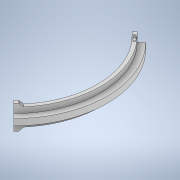
# Autodesk Inventor part: BinnenringMiddenStuk
Saved by Autodesk Inventor 2022 (Build 260153000, 153)
## iProperties
Created: 2022-04-04
Part Number: BinnenringMiddenStuk
Material: Generic
Document SubType Name: Modeling
Designer: Seppe
Density: 1 g/cm^3
Appearance: Default
Author: Seppe
Autodesk Inventor part; units mm, degrees
ref_plane "YZ Plane" through (0, 0, 0) normal (1, 0, 0) x (0, 1, 0)
sketch "Sketch1" plane through (0, 0, 0) normal (0, 1, 0) x (-1, 0, 0)
  circle A0 centre (0, 0) radius 124.6
  circle A1 centre (0, 0) radius 114.6
  line L0 (0, -124.6) -> (0, 124.6)
  point P0 (0, 114.6)
  point P1 (0, -114.6)
  dimension "d88" = 249.2
  dimension "d89" = 229.2
  constraints: 2 centre point, 2 end point, 2 point on circle, 1 coincident, 1 vertical
  measures "d88" diameter of A0
  measures "d89" diameter of A1
extrude "Extrusion18" add sketch "Sketch1" along normal mid plane 25 contours L0 A1 A0 picked at (-5.2055, 120.9392)
sketch "Sketch21" plane through (0, 0, 0) normal (0, 1, 0) x (-1, 0, 0)
  circle A0 centre (0, 0) radius 124.6
  circle A1 centre (0, 0) radius 133.25
  line L0 (0, -133.25) -> (0, 133.25)
  point P0 (0, -124.6)
  point P1 (0, 124.6)
  dimension "d92" = 266.5
  constraints: 2 centre point, 2 coincident, 2 end point, 2 point on circle, 1 vertical
  measures "d92" diameter of A1
extrude "Extrusion19" add sketch "Sketch21" along normal mid plane 9 contours A0 L0 A1 picked at (-127.3194, 0)
ref_plane "Work Plane2" through (0, 0, -114.6) normal (0, 0, 1) x (1, 0, 0)
sketch "Sketch23" plane through (0, 0, -114.6) normal (0, 0, 1) x (1, 0, 0)
  line L0 (0, 17.5) -> (6.5, 17.5)
  line L1 (6.5, 17.5) -> (6.5, -17.5)
  line L2 (6.5, -17.5) -> (0, -17.5)
  line L3 (0, -17.5) -> (0, 17.5)
  line L4 (0, -12.5) -> (0, 12.5) projected
  point P0 (0, 0)
  point P1 (0, 8)
  dimension "d98" = 6.5
  dimension "d99" = 35
  dimension "d100" = 0
  dimension "d101" = 17.5
  constraints: 8 end point, 2 parallel, 1 horizontal, 1 perpendicular
  measures "d98" distance of L1.end L2.end
  measures "d99" distance of L0.end L1.end
  measures "d100" distance between parallel lines of L4 L3
  measures "d101" distance from line of point (0, 0) L0
extrude "Extrusion21" add sketch "Sketch23" against normal blind 10
sketch "Sketch25" plane through (0, 0, 0) normal (0, 1, 0) x (-1, 0, 0)
  line L0 (0, -114.6) -> (-11.5, -114.6)
  line L1 (-11.5, -114.6) -> (-11.5, -104.6)
  line L2 (-11.5, -104.6) -> (0, -104.6)
  line L3 (0, -104.6) -> (0, -114.6)
  point P0 (0, 0)
  dimension "d104" = 11.5
  dimension "d105" = 10
  constraints: 8 end point, 2 parallel, 1 horizontal, 1 perpendicular
  measures "d104" distance of L1.end L2.end
  measures "d105" distance of L0.end L1.end
extrude "Extrusion22" cut sketch "Sketch25" along normal through all both and the other way through all
ref_plane "Work Plane3" through (0, 17.5, -119.6) normal (0, 0, -1) x (1, 0, 0)
sketch "Sketch26" plane through (0, 17.5, -119.6) normal (0, 0, -1) x (1, 0, 0)
  circle A0 centre (0, 17.5) radius 13
  dimension "d108" = 26
  constraints: 1 centre point, 1 coincident
  measures "d108" diameter of A0
extrude "Extrusion23" cut sketch "Sketch26" along normal mid plane 6
sketch "Sketch27" plane through (0, 17.5, -119.6) normal (0, 0, -1) x (1, 0, 0)
  circle A0 centre (0, 17.5) radius 8
  dimension "d111" = 16
  constraints: 1 centre point, 1 coincident
  measures "d111" diameter of A0
extrude "Extrusion24" cut sketch "Sketch27" along normal through all both and the other way through all
sketch "Sketch28" plane through (0, 4.5, 0) normal (0, 1, 0) x (1, 0, 0)
  line L0 (6.6144, 133.0857) -> (6.6144, 124.4243) projected
  circle A0 centre (33.7757, 0) radius 127.3544
  circle A1 centre (0, 0) radius 168.1211
  line L1 (-168.1211, 0) -> (168.1211, 0)
  line L2 (6.6144, 124.4243) -> (6.6144, 167.991)
  point P0 (161.1301, 0)
  constraints: 4 end point, 3 point on circle, 1 centre point, 1 coincident, 1 horizontal, 1 point on line, 3 other
extrude "Extrusion25" cut sketch "Sketch28" along normal through all both and the other way through all contours L2 A1 L1 A0 L0 picked at (33.6565, 152.3073)
sketch "Sketch29" plane through (0, 17.5, -124.6) normal (-1, 0, 0) x (0, 0, 1)
  circle A0 centre (2.5, -2.5) radius 1
  circle A1 centre (7.5, -2.5) radius 1
  circle A2 centre (2.5, -32.5) radius 1
  circle A3 centre (7.5, -32.5) radius 1
  line L0 (0, -9.5) -> (0, 0) projected
  line L1 (10, 0) -> (0, 0) projected
  line L2 (10, -9.5) -> (10, 0) projected
  line L3 (10, -35) -> (0, -35) projected
  line L4 (0, -35) -> (0, -25.5) projected
  line L5 (10, -35) -> (10, -25.5) projected
  point P0 (124.6, -17.5)
  dimension "d119" = 2
  dimension "d120" = 2
  dimension "d121" = 2
  dimension "d122" = 2
  dimension "d123" = 2.5
  dimension "d124" = 2.5
  dimension "d125" = 2.5
  dimension "d126" = 2.5
  dimension "d127" = 2.5
  dimension "d128" = 2.5
  dimension "d129" = 2.5
  dimension "d130" = 2.5
  constraints: 4 centre point
  measures "d119" diameter of A0
  measures "d120" diameter of A1
  measures "d121" diameter of A2
  measures "d122" diameter of A3
  measures "d123" distance from line of L0 A0.centre
  measures "d124" distance from line of L1 A0.centre
  measures "d125" distance from line of L1 A1.centre
  measures "d126" distance from line of L2 A1.centre
  measures "d127" distance from line of L3 A2.centre
  measures "d128" distance from line of L4 A2.centre
  measures "d129" distance from line of L3 A3.centre
  measures "d130" distance from line of L5 A3.centre
extrude "Extrusion26" cut sketch "Sketch29" against normal blind 6.5
sketch "Sketch31" plane through (0, 0, -124.6) normal (0, 0, -1) x (-1, 0, 0)
  line L0 (-6.5, 17.5) -> (-6.5, 4.6637) projected
  line L1 (-6.5, 12.5) -> (-11.5, 12.5) projected
  line L2 (-6.5, 17.5) -> (-11.5, 17.5)
  line L3 (-11.5, 17.5) -> (-11.5, 12.5)
  line L4 (-11.5, 12.5) -> (-6.5, 12.5)
  line L5 (-6.5, 12.5) -> (-6.5, 17.5)
  line L6 (-11.5, 12.5) -> (-6.5, 17.5)
  point P0 (0, 0)
  constraints: 10 end point, 2 parallel, 1 horizontal, 1 perpendicular
extrude "Extrusion28" add sketch "Sketch31" against normal blind 10 contours L0 L1 L6
sketch "Sketch33" plane through (6.5, 15, -122.1) normal (-1, 0, 0) x (0, 0, 1)
  circle A0 centre (0, 0) radius 2
  circle A1 centre (5, 0) radius 1 projected
  circle A2 centre (5, 0) radius 2
  circle A3 centre (0, -30) radius 1 projected
  circle A4 centre (0, -30) radius 2
  circle A5 centre (5, -30) radius 1 projected
  circle A6 centre (5, -30) radius 2
  point P0 (122.1, -15)
  dimension "d137" = 4
  dimension "d138" = 4
  dimension "d139" = 4
  dimension "d140" = 4
  constraints: 4 centre point, 3 coincident
  measures "d137" diameter of A0
  measures "d138" diameter of A2
  measures "d139" diameter of A4
  measures "d140" diameter of A6
extrude "Extrusion29" cut sketch "Sketch33" against normal blind 10 contours A0 | A1 | A2 | A3 | A4 | A5 | A6
sketch "Sketch34" plane through (0, 12.5, 0) normal (0, 1, 0) x (1, 0, 0)
  circle A0 centre (0, 0) radius 124.6
  circle A1 centre (0, 0) radius 133.25
  constraints: 2 centre point, 2 coincident
extrude "Extrusion30" cut sketch "Sketch34" along normal blind 5 and the other way blind 8
mirror "Mirror1" about plane through (0, 0, 0) normal (0, 1, 0) of "Extrusion29", "Extrusion26", "Extrusion28"
sketch "Sketch35" plane through (0, -12.5, 0) normal (0, -1, 0) x (1, 0, 0)
  circle A0 centre (0, 0) radius 124.6
  arc A1 (11.5, -124.0682) -> (0, 124.6) centre (0, 0) ccw projected
  circle A2 centre (0, 0) radius 127.0013
  constraints: 2 centre point, 2 coincident
extrude "Extrusion31" cut sketch "Sketch35" along normal blind 5 and the other way blind 8
mirror "Mirror2" about plane through (0, 0, 0) normal (0, 0, 1) of "Extrusion29", "Extrusion28", "Extrusion21", "Extrusion24", "Extrusion23", "Extrusion26"
mirror "Mirror3" about plane through (0, 0, 0) normal (0, 0, 1) of "Extrusion25"
mirror "Mirror4" about plane through (0, 0, 0) normal (0, 0, 1) of "Extrusion30"
sketch "Sketch37" plane through (0, 12.5, 0) normal (0, 1, 0) x (1, 0, 0)
  line L0 (6.5, -114.6) -> (0, -114.6) projected
  line L1 (0, -114.6) -> (11.5, -114.6)
  line L2 (11.5, -114.6) -> (11.5, -107.0167)
  line L3 (11.5, -107.0167) -> (0, -107.0167)
  line L4 (0, -107.0167) -> (0, -114.6)
  point P0 (0, 0)
  constraints: 8 end point, 2 parallel, 1 horizontal, 1 perpendicular
extrude "Extrusion32" cut sketch "Sketch37" against normal through all
sketch "Sketch42" plane through (0, 12.5, 0) normal (0, 1, 0) x (1, 0, 0)
  line L0 (0, 0) -> (94.222, -94.222)
  arc A0 (39.6322, -127.2197) -> (39.6322, 127.2197) centre (0, 0) ccw projected
  line L1 (0, 0) -> (133.25, 0) construction
  circle A1 centre (0, 0) radius 124.6
  circle A2 centre (0, 0) radius 114.6
  arc A3 (11.5, -124.0682) -> (11.5, 124.0682) centre (0, 0) ccw projected
  arc A4 (11.5, -114.0215) -> (11.5, 114.0215) centre (0, 0) ccw projected
  line L2 (88.1055, -88.1055) -> (81.0344, -81.0344)
  line L3 (81.0344, -81.0344) -> (77.4989, -84.57)
  line L4 (77.4989, -84.57) -> (84.57, -91.641)
  line L5 (84.57, -91.641) -> (88.1055, -88.1055)
  line L6 (88.1055, -88.1055) -> (81.0344, -81.0344)
  line L7 (81.0344, -81.0344) -> (84.57, -77.4989)
  line L8 (84.57, -77.4989) -> (91.641, -84.57)
  line L9 (91.641, -84.57) -> (88.1055, -88.1055)
  line L10 (0, 0) -> (88.1055, 88.1055)
  line L11 (81.0344, 81.0344) -> (88.1055, 88.1055)
  line L12 (88.1055, 88.1055) -> (84.57, 91.641)
  line L13 (84.57, 91.641) -> (77.4989, 84.57)
  line L14 (77.4989, 84.57) -> (81.0344, 81.0344)
  line L15 (81.0344, 81.0344) -> (88.1055, 88.1055)
  line L16 (88.1055, 88.1055) -> (91.641, 84.57)
  line L17 (91.641, 84.57) -> (84.57, 77.4989)
  line L18 (84.57, 77.4989) -> (81.0344, 81.0344)
  point P0 (91.5701, 84.499)
  point P1 (84.499, 91.5701)
  point P2 (91.5701, -84.499)
  point P3 (84.499, -91.5701)
  dimension "d164" = 45
  dimension "d165" = 5
  dimension "d166" = 5
  dimension "d167" = 5
  dimension "d168" = 5
  constraints: 38 end point, 8 parallel, 5 point on circle, 4 perpendicular, 3 collinear, 3 point on line, 2 centre point, 2 coincident, 1 equal length, 1 horizontal
  measures "d164" angle of L0 L1
  measures "d165" distance of L3.end L2.end
  measures "d166" distance of L2.end L7.end
  measures "d167" distance of L12.end L10.end
  measures "d168" distance of L10.end L16.end
extrude "Extrusion33" add sketch "Sketch42" along normal blind 5 contours L7 L8 A1 L0 | L0 A1 L4 L3 | L14 L13 A1 L10 | L10 A1 L17 L18
sketch "Sketch45" plane through (0, 0, 0) normal (0, 1, 0) x (-1, 0, 0)
  circle A0 centre (0, 0) radius 119.6
  line L0 (0, 0) -> (-12.1737, 118.9788)
  line L1 (0, 0) -> (-133.25, 0)
  arc A1 (-39.6322, 127.2197) -> (-39.6322, -127.2197) centre (0, 0) ccw projected
  line L2 (0, 0) -> (-12.1737, -118.9788)
  dimension "d171" = 239.2
  dimension "d172" = 119.6
  constraints: 6 end point, 1 centre point, 1 coincident, 1 horizontal, 1 point on circle, 1 symmetric about line
  measures "d171" diameter of A0
  measures "d172" distance of L0.start L0.end
extrude "Extrusion34" cut sketch "Sketch45" along normal through all both and the other way through all contours L0 L1 A0 | A0 L1 L2
sketch "Sketch46" plane through (0, 12.5, 0) normal (0, 1, 0) x (1, 0, 0)
  line L0 (11.5, -114.6) -> (6.5, -114.6) projected
  line L1 (11.5, -114.6) -> (34.9222, -114.6)
  line L2 (34.9222, -114.6) -> (34.9222, -118.5669)
  line L3 (34.9222, -118.5669) -> (11.5, -118.5669)
  line L4 (11.5, -118.5669) -> (11.5, -114.6)
  line L5 (11.5, -114.6) -> (11.5, -124.0682) projected
  line L6 (18.8955, -118.5669) -> (11.5, -118.5669)
  line L7 (11.5, -118.5669) -> (11.5, -120.4367)
  line L8 (11.5, -120.4367) -> (18.8955, -120.4367)
  line L9 (18.8955, -120.4367) -> (18.8955, -118.5669)
  point P0 (0, 0)
  constraints: 16 end point, 4 parallel, 2 horizontal, 2 perpendicular, 2 point on line
extrude "Extrusion35" add sketch "Sketch46" against normal blind 25
sketch "Sketch47" plane through (0, 12.5, 0) normal (0, 1, 0) x (1, 0, 0)
  line L0 (11.5, -114.6) -> (11.5, -114.0215) projected
  line L1 (11.5, -114.6) -> (11.5, -114.0215)
  arc A0 (11.5, -114.0215) -> (11.6648, -114.0048) centre (0, 0) ccw projected
  line L2 (11.5, -114.0215) -> (11.6648, -114.0048)
  line L3 (11.6648, -114.0048) -> (11.7257, -114.6) projected
  line L4 (11.6648, -114.0048) -> (11.7257, -114.6)
  line L5 (6.5, -114.6) -> (11.5, -114.6) projected
  line L6 (11.7257, -114.6) -> (11.5, -114.6)
  constraints: 8 end point, 3 collinear
extrude "Extrusion36" cut sketch "Sketch47" against normal blind 25
sketch "Sketch48" plane through (0, 0, 116.6) normal (0, 0, 1) x (1, 0, 0)
  circle A0 centre (0, 0) radius 13
  constraints: 1 centre point, 1 coincident
extrude "Extrusion37" cut sketch "Sketch48" along normal blind 6
sketch "Sketch49" plane through (84.499, 12.5, -91.5701) normal (-0.7071068, 0, -0.7071068) x (-0.7071068, 0, 0.7071068)
  circle A0 centre (2.5042, 2.5) radius 1
  line L0 (0, 5) -> (5.0042, 5) projected
  line L1 (5.0042, 0) -> (5.0042, 5) projected
  point P0 (124.4996, -12.5)
  dimension "d181" = 2
  dimension "d182" = 2.5
  dimension "d183" = 2.5
  constraints: 1 centre point
  measures "d181" diameter of A0
  measures "d182" distance from line of L0 A0.centre
  measures "d183" distance from line of L1 A0.centre
extrude "Extrusion38" cut sketch "Sketch49" against normal through all
sketch "Sketch50" plane through (84.499, 12.5, 91.5701) normal (-0.7071068, 0, 0.7071068) x (0.7071068, 0, 0.7071068)
  circle A0 centre (-2.5, 2.5) radius 1
  line L0 (-5.0042, 5) -> (0, 5) projected
  line L1 (0, 0) -> (0, 5) projected
  point P0 (-124.4996, -12.5)
  dimension "d186" = 2
  dimension "d187" = 2.5
  dimension "d188" = 2.5
  constraints: 1 centre point
  measures "d186" diameter of A0
  measures "d187" distance from line of L0 A0.centre
  measures "d188" distance from line of L1 A0.centre
extrude "Extrusion39" cut sketch "Sketch50" against normal blind 10
mirror "Mirror6" about plane through (0, 0, 0) normal (0, 0, 1) of "Extrusion35", "Extrusion36", "Extrusion37"
sketch "Sketch38" plane through (0, 0, 0) normal (0, 1, 0) x (-1, 0, 0)
  line L0 (0, 0) -> (-94.222, -94.222)
  arc A0 (-39.6322, 127.2197) -> (-39.6322, -127.2197) centre (0, 0) ccw projected
  line L1 (0, 0) -> (133.25, 0) construction
  line L2 (0, 0) -> (-94.222, 94.222)
  line L3 (0, 0) -> (133.25, 0) construction
  circle A1 centre (0, 0) radius 133.25
  point P0 (-39.6322, -127.2197)
  dimension "d156" = 135
  dimension "d157" = 225
  constraints: 8 end point, 2 equal length, 2 horizontal, 2 point on circle, 1 centre point, 1 coincident
  measures "d156" angle of L0 L1
mirror "Mirror7" about plane through (0, 0, 0) normal (0, 1, 0) of "Extrusion33", "Extrusion39", "Extrusion38"
sketch "Sketch51" plane through (0, -17.5, 0) normal (0, -1, 0) x (0.7071068, 0, 0.7071068)
  line L0 (-5, -114.6) -> (5, -114.6) projected
  line L1 (-5, -114.6) -> (5, -114.6)
  line L2 (5, -114.6) -> (5, -119.4954)
  line L3 (-5, -119.4954) -> (-5, -114.6)
  line L4 (124.4996, -5) -> (114.6, -5) projected
  line L5 (114.6, -5) -> (114.6, 5) projected
  line L6 (114.6, -5) -> (114.6, 5)
  line L7 (114.6, 5) -> (119.4954, 5)
  line L8 (119.4954, -5) -> (114.6, -5)
  arc A0 (-5, -119.4954) -> (5, -119.4954) centre (0, 0) ccw projected
  arc A1 (5, -119.4954) -> (0, -119.6) centre (0, 0) ccw
  arc A2 (119.4954, -5) -> (119.4954, 5) centre (0, 0) ccw projected
  arc A3 (5, -119.4954) -> (119.4954, -5) centre (0, 0) ccw projected
  arc A4 (119.6, 0) -> (119.4954, -5) centre (0, 0) ccw
  point P0 (119.4954, -5)
  constraints: 12 end point, 8 point on circle, 4 equal length, 2 centre point, 2 perpendicular
extrude "Extrusion40" cut sketch "Sketch51" against normal blind 10 contours L0 L2 A0 L3 | A1 L4 L5 L7
extrude "Extrusion41" cut sketch "Sketch38" along normal through all both and the other way through all contours L2 A0 A1 L0
sketch "Sketch53" plane through (0, 12.5, 0) normal (0, 1, 0) x (1, 0, 0)
  line L0 (88.0316, 80.9605) -> (91.5701, 84.499) projected
  line L1 (88.0316, 80.9605) -> (91.5701, 84.499)
  line L2 (91.5701, 84.499) -> (95.1056, 80.9635)
  line L3 (95.1056, 80.9635) -> (91.5671, 77.425)
  line L4 (91.5671, 77.425) -> (88.0316, 80.9605)
  arc A0 (88.0316, -80.9605) -> (88.0316, 80.9605) centre (0, 0) ccw projected
  line L5 (91.5701, -84.499) -> (88.0316, -80.9605) projected
  line L6 (88.0316, -80.9605) -> (91.5701, -84.499)
  line L7 (91.5701, -84.499) -> (95.1056, -80.9635)
  line L8 (95.1056, -80.9635) -> (91.5671, -77.425)
  line L9 (91.5671, -77.425) -> (88.0316, -80.9605)
  circle A1 centre (0, 0) radius 124.6
  circle A2 centre (0, 0) radius 119.6
  arc A3 (88.1055, -88.1055) -> (88.1055, 88.1055) centre (0, 0) ccw projected
  line L10 (94.8924, -80.7502) -> (91.3449, -77.2028)
  line L11 (94.8924, 80.7502) -> (91.3449, 77.2028)
  point P0 (94.8924, -80.7502)
  dimension "d195" = 5
  dimension "d198" = 5
  constraints: 20 end point, 6 equal length, 4 point on circle, 4 point on line, 2 centre point, 2 coincident, 2 perpendicular, 1 concentric
  measures "d195" distance of L0.end L2.end
  measures "d198" distance of L7.end L5.start
extrude "Extrusion42" add sketch "Sketch53" along normal blind 5 contours L0 A1 L3 L4 | L4 L11 A0 | L9 L8 A1 L5 | A0 L10 L9
chamfer "Chamfer2" distance 5 angle 45 2 edges at (93.1186, 17.5, 78.9765) (93.1186, 17.5, -78.9765)
sketch "Sketch54" plane through (89.7993, 15, -82.7283) normal (-0.7071068, 0, -0.7071068) x (-0.7071068, 0, 0.7071068)
  circle A0 centre (0, 0) radius 2
  point P0 (121.9954, -15)
  dimension "d202" = 4
  constraints: 1 centre point
  measures "d202" diameter of A0
extrude "Extrusion43" cut sketch "Sketch54" against normal blind 5
sketch "Sketch55" plane through (89.8023, 15, 82.7312) normal (-0.7071068, 0, 0.7071068) x (0.7071068, 0, 0.7071068)
  circle A0 centre (0, 0) radius 2
  point P0 (-121.9996, -15)
  dimension "d205" = 4
  constraints: 1 centre point
  measures "d205" diameter of A0
extrude "Extrusion44" cut sketch "Sketch55" against normal blind 5
mirror "Mirror8" about plane through (0, 0, 0) normal (0, 1, 0) of "Extrusion42", "Chamfer2", "Extrusion43", "Extrusion44", "Extrusion39"
equation "\"d125\" = d124"
equation "\"d126\" = d123"
body "Solid3"
